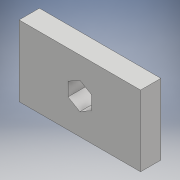
# Autodesk Inventor part: jalador
Saved by Autodesk Inventor 2018.3 (Build 223284000, 284)
## iProperties
Created: 2019-02-25
Part Number: jalador
Material: Generic
Document SubType Name: Modeling
Designer: Mario
Density: 1 g/cm^3
Appearance: Default
Author: Mario
Autodesk Inventor part; units mm, degrees
ref_plane "YZ Plane" through (0, 0, 0) normal (1, 0, 0) x (0, 1, 0)
ref_plane "XZ Plane" through (0, 0, 0) normal (0, 1, 0) x (-1, 0, 0)
ref_plane "XY Plane" through (0, 0, 0) normal (0, 0, 1) x (1, 0, 0)
sketch "Sketch1" plane through (0, 0, 0) normal (0, 1, 0) x (-1, 0, 0)
  line L0 (14.9498, 8.7133) -> (-14.9498, 8.7133)
  line L1 (-14.9498, 8.7133) -> (-14.9498, -8.7133)
  line L2 (-14.9498, -8.7133) -> (14.9498, -8.7133)
  line L3 (14.9498, -8.7133) -> (14.9498, 8.7133)
  line L4 (14.9498, 8.7133) -> (-14.9498, -8.7133) construction
  line L5 (-14.9498, 8.7133) -> (14.9498, -8.7133) construction
  point P0 (0, 0)
  constraints: 12 end point, 2 midpoint, 2 parallel, 1 horizontal, 1 perpendicular
extrude "Extrusion1" add sketch "Sketch1" along normal blind 5
sketch "Sketch2" plane through (0, 5, 0) normal (0, 1, 0) x (1, 0, 0)
  line L0 (-2.9037, 1.6764) -> (0, 3.3529)
  line L1 (0, 3.3529) -> (2.9037, 1.6764)
  line L2 (2.9037, 1.6764) -> (2.9037, -1.6764)
  line L3 (2.9037, -1.6764) -> (0, -3.3529)
  line L4 (0, -3.3529) -> (-2.9037, -1.6764)
  line L5 (-2.9037, -1.6764) -> (-2.9037, 1.6764)
  point P0 (0, 0)
  point P1 (0, 0)
  constraints: 12 end point, 1 coincident, 1 vertical, 13 other
extrude "Extrusion2" cut sketch "Sketch2" against normal blind 5
body "Solid1"
